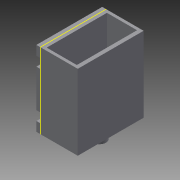
# Autodesk Inventor part: atmos-pressure-end
Saved by Autodesk Inventor 2014 SP2 (Build 180246200, 246)
## iProperties
Created: 2014-06-30
Part Number: atmos-pressure-end
Material: Generic
Document SubType Name: Modeling
Designer: pjb08r
Density: 1 g/cm^3
Appearance: Default
Author: pjb08r
Autodesk Inventor part; units mm, degrees
ref_plane "YZ Plane" through (0, 0, 0) normal (1, 0, 0) x (0, 1, 0)
ref_plane "XZ Plane" through (0, 0, 0) normal (0, 1, 0) x (-1, 0, 0)
ref_plane "XY Plane" through (0, 0, 0) normal (0, 0, 1) x (1, 0, 0)
sketch "Sketch1" plane through (0, 0, 0) normal (0, 0, 1) x (1, 0, 0)
  line L0 (-10, -17.5) -> (10, -17.5)
  line L1 (10, -17.5) -> (10, 17.5)
  line L2 (10, 17.5) -> (-10, 17.5)
  line L3 (-10, 17.5) -> (-10, -17.5)
  line L4 (-10, -17.5) -> (10, 17.5) construction
  line L5 (10, -17.5) -> (-10, 17.5) construction
  point P0 (0, 0)
  dimension "d0" = 20
  dimension "d1" = 35
  constraints: 12 end point, 2 midpoint, 2 parallel, 1 horizontal, 1 perpendicular
  measures "d0" distance of L2.end L1.end
  measures "d1" distance of L1.end L0.end
extrude "Extrusion1" add sketch "Sketch1" along normal blind 40
sketch "Sketch2" plane through (0, 0, 40) normal (0, 0, 1) x (1, 0, 0)
  line L0 (-8, -16) -> (8, -16)
  line L1 (8, -16) -> (8, 16)
  line L2 (8, 16) -> (-8, 16)
  line L3 (-8, 16) -> (-8, -16)
  point P0 (0, 0)
  dimension "d4" = 16
  dimension "d5" = 32
  constraints: 8 end point, 2 parallel, 1 horizontal, 1 perpendicular
  measures "d4" distance of L2.end L1.end
  measures "d5" distance of L1.end L0.end
extrude "Extrusion2" cut sketch "Sketch2" against normal blind 30
sketch "Sketch3" plane through (0, 0, 10) normal (0, 0, 1) x (1, 0, 0)
  line L0 (8, -16) -> (-8, -16) projected
  line L1 (8, 16) -> (8, -16) projected
  line L2 (-8, 16) -> (8, 16) projected
  line L3 (-8, -16) -> (-8, 16) projected
  point P0 (0, 0)
sketch "Sketch5" plane through (-10, -17.5, 0) normal (-1, 0, 0) x (0, 0, 1)
  line L0 (0, 35) -> (0, 0) projected
  line L1 (0, 0) -> (40, 0) projected
  line L2 (40, 35) -> (40, 0) projected
  line L3 (0, 35) -> (40, 35) projected
  point P0 (0, 17.5)
sketch "Sketch6" plane through (-10, -17.5, 0) normal (-1, 0, 0) x (0, 0, 1)
  line L0 (0, 35) -> (0, 0) projected
  line L1 (0, 0) -> (40, 0) projected
  line L2 (0, 35) -> (40, 35) projected
  line L3 (0, 35) -> (5, 35)
  line L4 (5, 35) -> (5, 0)
  line L5 (5, 0) -> (0, 0)
  line L6 (0, 0) -> (0, 35)
  line L7 (40, 35) -> (35, 35)
  line L8 (35, 35) -> (35, 0)
  line L9 (35, 0) -> (40, 0)
  line L10 (40, 0) -> (40, 35)
  line L11 (10, 0) -> (30, 0)
  line L12 (30, 0) -> (30, 35)
  line L13 (30, 35) -> (10, 35)
  line L14 (10, 35) -> (10, 0)
  point P0 (0, 17.5)
  dimension "d16" = 5
  dimension "d17" = 5
  dimension "d18" = 20
  constraints: 24 end point, 6 parallel, 4 point on line, 3 horizontal, 3 perpendicular
  measures "d16" distance of L4.end L5.end
  measures "d17" distance of L9.end L8.end
  measures "d18" distance of L13.end L12.end
extrude "Extrusion3" add sketch "Sketch6" along normal blind 2 contours L2 L4 L1 L0 | L2 L12 L1 L14 | L2 L10 L1 L8
sketch "Sketch7" plane through (0, 0, 10) normal (0, 0, 1) x (1, 0, 0)
  circle A0 centre (0, 4) radius 2.25
  point P0 (0, 0)
  dimension "d21" = 4.5
  constraints: 1 centre point
  measures "d21" diameter of A0
extrude "Extrusion4" cut sketch "Sketch7" against normal through all
sketch "Sketch8" plane through (0, 0, 0) normal (0, 0, -1) x (-1, 0, 0)
  circle A0 centre (0, 4) radius 2.25 projected
  circle A1 centre (0, 4) radius 3.5
  point P0 (0, 0)
  dimension "d24" = 7
  constraints: 1 centre point, 1 coincident
  measures "d24" diameter of A1
extrude "Extrusion5" add sketch "Sketch8" along normal blind 8
body "Solid1"
